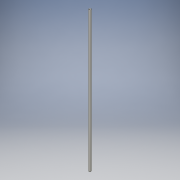
# Autodesk Inventor part: RSHC10XX00 Rack (Simplified)-58
Saved by Autodesk Inventor 2018.2 (Build 222227000, 227)
## iProperties
Created: 2018-01-21
Part Number: RSHC10XX00 Rack (Simplified)-58
Material: Steel
Document SubType Name: Modeling
Designer: torba
Density: 7.85 g/cm^3
Appearance: Steel
Author: torba
Autodesk Inventor part; units mm, degrees
ref_plane "YZ Plane" through (0, 0, 0) normal (1, 0, 0) x (0, 1, 0)
ref_plane "XZ Plane" through (0, 0, 0) normal (0, 1, 0) x (-1, 0, 0)
ref_plane "XY Plane" through (0, 0, 0) normal (0, 0, 1) x (1, 0, 0)
sketch "Sketch1" plane through (0, 0, 0) normal (0, 1, 0) x (-1, 0, 0)
  line L0 (0, 0) -> (15, 0)
  line L1 (15, 0) -> (15, -14)
  line L2 (15, -14) -> (0, -14)
  line L3 (0, -14) -> (0, 0)
  dimension "d0" = 15
  dimension "d1" = 14
  constraints: 8 end point, 2 parallel, 1 horizontal, 1 perpendicular
  measures "d0" distance of L1.end L2.end
  measures "d1" distance of L0.end L1.end
extrude "Extrusion1" add sketch "Sketch1" along normal blind 1473.2
sketch "Sketch2" plane through (0, 0, 0) normal (0, 0, 1) x (1, 0, 0)
  line L0 (0, 0) -> (-15, 0) projected
  line L1 (0, 0) -> (0, 1473.2) projected
  line L2 (-15, 1473.2) -> (0, 1473.2) projected
  line L3 (-15, 0) -> (-15, 1473.2) projected
extrude "Extrusion2" add sketch "Sketch2" along normal blind 2 separate body
body "Solid1"
body "Solid2"
